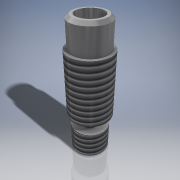
# Autodesk Inventor part: HeatBreak
Saved by Autodesk Inventor 2019 (Build 230136000, 136)
## iProperties
Created: 2021-03-14
Part Number: HeatBreak
Material: Générique
Document SubType Name: Modeling
Designer: thoma
Density: 1 g/cm^3
Appearance: Acier
Author: thoma
Autodesk Inventor part; units mm, degrees
ref_plane "YZ Plane" through (0, 0, 0) normal (1, 0, 0) x (0, 1, 0)
ref_plane "XZ Plane" through (0, 0, 0) normal (0, 1, 0) x (-1, 0, 0)
ref_plane "XY Plane" through (0, 0, 0) normal (0, 0, 1) x (1, 0, 0)
sketch "Esquisse1" plane through (0, 0, 0) normal (1, 0, 0) x (0, 1, 0)
  line L0 (0, 0) -> (0, -3)
  line L1 (0, -3) -> (-4.5, -3)
  line L2 (-4.5, -3) -> (-4.5, -3.5)
  line L3 (-4.5, -3.5) -> (-15, -3.5)
  line L4 (0, 0) -> (-22.1, 0)
  line L5 (-22.1, 0) -> (-22.1, -3)
  line L6 (-22.1, -3) -> (-17.1, -3)
  line L7 (-15.8588, 0) -> (-15.8588, -1) construction
  line L8 (-15.8588, -1) -> (-15.8588, -1.48) construction
  line L9 (-17.1, -3) -> (-17.1, -1.48)
  line L10 (-17.1, -1.48) -> (-15, -1.48)
  line L11 (-15, -1.48) -> (-15, -3.5)
  dimension "d0" = 3
  dimension "d1" = 4.5
  dimension "d2" = 0.5
  dimension "d3" = 10.5
  dimension "d4" = 22.1
  dimension "d5" = 3
  dimension "d6" = 5
  dimension "d7" = 1
  dimension "d8" = 0.48
  constraints: 24 end point, 6 perpendicular, 4 vertical, 2 point on line, 1 horizontal
  measures "d0" distance of L0.start L0.end
  measures "d1" distance of L0.end L1.end
  measures "d2" distance of L1.end L2.end
  measures "d3" distance of L2.end L3.end
  measures "d4" distance of L0.start L4.end
  measures "d5" distance of L4.end L5.end
  measures "d6" distance of L5.end L6.end
  measures "d7" distance of L7.start L7.end
  measures "d8" distance of L7.end L8.end
revolve "Révolution1" add sketch "Esquisse1" angle 360 about axis through (0, 0, 0) along (0, -1, 0)
sketch "Esquisse2" plane through (0, 0, 0) normal (0, 1, 0) x (1, 0, 0)
  circle A0 centre (0, 0) radius 1
  dimension "d10" = 2
  constraints: 1 centre point, 1 coincident
  measures "d10" diameter of A0
extrude "Extrusion1" cut sketch "Esquisse2" against normal up to next
sketch "Esquisse3" plane through (0, 0, 0) normal (0, 1, 0) x (1, 0, 0)
  circle A0 centre (0, 0) radius 3 projected
  circle A1 centre (0, 0) radius 2.05
  dimension "d13" = 4.1
  constraints: 1 centre point, 1 coincident
  measures "d13" diameter of A1
extrude "Extrusion2" cut sketch "Esquisse3" against normal up to surface (4.5 mm away) contours A1
chamfer "Chanfrein1" distance 0.5 angle 45 1 edges at (-1, -4.5, 0)
chamfer "Chanfrein2" distance 0.5 angle 45 1 edges at (0, -22.1, 3)
chamfer "Chanfrein3" distance 0.5 angle 45 1 edges at (0, 0, 3)
thread "Filetage1" size "M7x1" class "6g" standard "ANSI Metric M Profile" full length
thread "Filetage2" size "M6x1" class "6g" standard "ANSI Metric M Profile" full length
